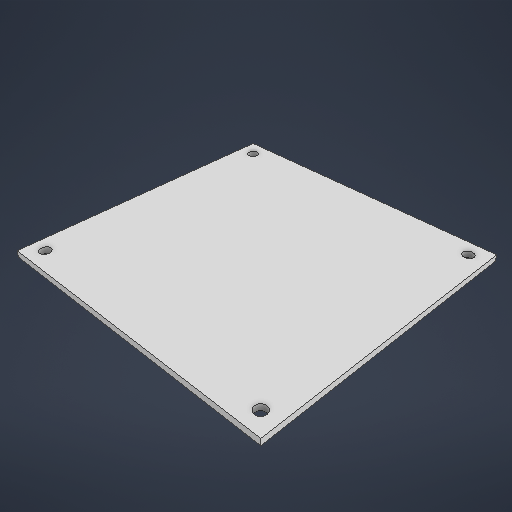
# Autodesk Inventor part: Case_Top
Saved by Autodesk Inventor 2026.1 (Build 301233000, 233)
## iProperties
Created: 2025-12-06
Part Number: Case_Top
Material: Generic
Document SubType Name: Modeling
Designer: chest
Density: 1 g/cm^3
Appearance: Default
Author: chest
Autodesk Inventor part; units mm, degrees
ref_plane "YZ Plane" through (0, 0, 0) normal (1, 0, 0) x (0, 1, 0)
ref_plane "XZ Plane" through (0, 0, 0) normal (0, 1, 0) x (-1, 0, 0)
ref_plane "XY Plane" through (0, 0, 0) normal (0, 0, 1) x (1, 0, 0)
sketch "Sketch1" plane through (0, 0, 0) normal (0, 1, 0) x (-1, 0, 0)
  line L0 (10.136, 16.6006) -> (-75.904, 16.6006)
  line L1 (-75.904, 16.6006) -> (-75.904, -66.8994)
  line L2 (-75.904, -66.8994) -> (10.136, -66.8994)
  line L3 (10.136, -66.8994) -> (10.136, 16.6006)
  point P0 (0, 0)
  dimension "d0" = 86.04
  dimension "d1" = 83.5
  constraints: 8 end point, 2 parallel, 1 horizontal, 1 perpendicular
  measures "d0" distance of L2.end L1.end
  measures "d1" distance of L1.end L0.end
extrude "Extrusion1" add sketch "Sketch1" along normal blind 2
sketch "Sketch2" plane through (0, 2, 0) normal (0, 1, 0) x (1, 0, 0)
  circle A0 centre (-5.136, -11.6006) radius 1.7
  line L0 (-10.136, 66.8994) -> (-10.136, -16.6006) projected
  line L1 (-10.136, -16.6006) -> (75.904, -16.6006) projected
  circle A1 centre (70.904, -11.6006) radius 1.7
  line L2 (75.904, -16.6006) -> (75.904, 66.8994) projected
  circle A2 centre (70.904, 61.8994) radius 1.7
  line L3 (75.904, 66.8994) -> (-10.136, 66.8994) projected
  circle A3 centre (-5.136, 61.8994) radius 1.7
  point P0 (0, 0)
  dimension "d4" = 3.4
  dimension "d5" = 5
  dimension "d6" = 5
  dimension "d7" = 3.4
  dimension "d8" = 5
  dimension "d9" = 5
  dimension "d10" = 3.4
  dimension "d11" = 5
  dimension "d12" = 5
  dimension "d13" = 3.4
  dimension "d14" = 5
  dimension "d15" = 5
  constraints: 4 centre point
  measures "d4" diameter of A0
  measures "d5" distance from line of L0 A0.centre
  measures "d6" distance from line of L1 A0.centre
  measures "d7" diameter of A1
  measures "d8" distance from line of L1 A1.centre
  measures "d9" distance from line of L2 A1.centre
  measures "d10" diameter of A2
  measures "d11" distance from line of L2 A2.centre
  measures "d12" distance from line of L3 A2.centre
  measures "d13" diameter of A3
  measures "d14" distance from line of L3 A3.centre
  measures "d15" distance from line of L0 A3.centre
extrude "Extrusion2" cut sketch "Sketch2" against normal blind 2 contours A0 | A1 | A2 | A3
body "Solid1"
